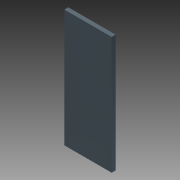
# Autodesk Inventor part: Lead Box Cover
Saved by Autodesk Inventor 2015 (Build 190159000, 159)
## iProperties
Created: 2015-03-10
Part Number: Lead Box Cover
Material: Lead
Document SubType Name: Modeling
Designer: pltwe4
Density: 11.34 g/cm^3
Appearance: Lead
Author: pltwe4
Autodesk Inventor part; units mm, degrees
ref_plane "YZ Plane" through (0, 0, 0) normal (1, 0, 0) x (0, 1, 0)
ref_plane "XZ Plane" through (0, 0, 0) normal (0, 1, 0) x (-1, 0, 0)
ref_plane "XY Plane" through (0, 0, 0) normal (0, 0, 1) x (1, 0, 0)
sketch "Sketch1" plane through (0, 0, 0) normal (0, 1, 0) x (-1, 0, 0)
  line L0 (-19.0875, -47.3815) -> (19.0875, -47.3815)
  line L1 (19.0875, -47.3815) -> (19.0875, 47.3815)
  line L2 (19.0875, 47.3815) -> (-19.0875, 47.3815)
  line L3 (-19.0875, 47.3815) -> (-19.0875, -47.3815)
  line L4 (-19.0875, -47.3815) -> (19.0875, 47.3815) construction
  line L5 (19.0875, -47.3815) -> (-19.0875, 47.3815) construction
  point P0 (0, 0)
  dimension "d0" = 94.763
  dimension "d1" = 38.175
  constraints: 12 end point, 2 midpoint, 2 parallel, 1 horizontal, 1 perpendicular
  measures "d0" distance of L0.end L1.end
  measures "d1" distance of L1.end L2.end
extrude "Extrusion1" add sketch "Sketch1" along normal blind 3.175
body "Solid1"
